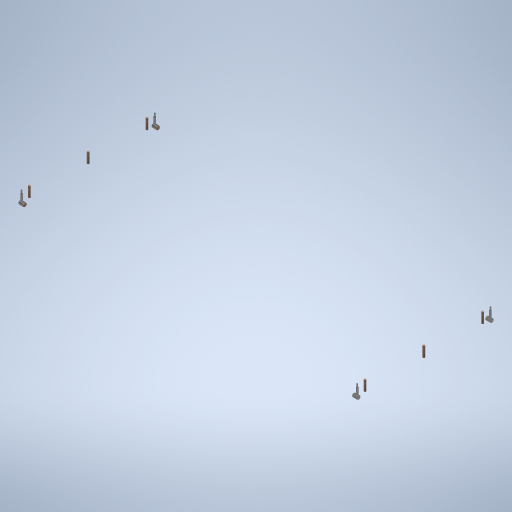
# Autodesk Inventor part: Minifixes pull Top Board-01
Saved by Autodesk Inventor 2024.3 (Build 283343000, 343)
## iProperties
RuleStatus: InUse
Created: 2014-05-13
Part Number: Minifixes pull Top Board-01
Material: Generic
Document SubType Name: Modeling
Designer: SauliusD
Density: 1 g/cm^3
Appearance: Default
Description: Minifixes pull Top Board
AfterDocNew0: Fire Form
Author: SauliusD
Autodesk Inventor part; units mm, degrees
ref_plane "XY Plane" through (0, 0, 0) normal (0, 0, 1) x (1, 0, 0)
sketch "Sketch1" plane through (0, 0, 0) normal (0, 0, 1) x (1, 0, 0)
  line L0 (-198.9585, 723.2553) -> (1147.0415, 723.2553)
  line L1 (1147.0415, 723.2553) -> (1147.0415, 177.2553)
  line L2 (1147.0415, 177.2553) -> (-198.9585, 177.2553)
  line L3 (-198.9585, 177.2553) -> (-198.9585, 723.2553)
  point P0 (0, 0)
  point P1 (474.0415, 177.2553)
  point P2 (-198.9585, 450.2553)
  constraints: 8 end point, 2 midpoint, 2 parallel, 1 horizontal, 1 perpendicular
ref_plane "Work Plane2" through (474.0415, 177.2553, 0) normal (1, 0, 0) x (0, 1, 0)
ref_plane "Work Plane3" through (-198.9585, 450.2553, 0) normal (0, 1, 0) x (-1, 0, 0)
sketch "Sketch3" plane through (0, 0, 0) normal (0, 0, 1) x (1, 0, 0)
  line L0 (-198.9585, 177.2553) -> (-198.9585, 723.2553) construction
  line L1 (-491.2585, 450.2553) -> (1439.3415, 450.2553) construction
  line L2 (474.0415, 897.0092) -> (474.0415, -298.2679) construction
  circle A0 centre (-211.4585, 178.2553) radius 4
  circle A1 centre (-211.4585, 210.2553) radius 4
  circle A2 centre (-211.4585, 722.2553) radius 4
  circle A3 centre (-211.4585, 690.2553) radius 4
  circle A4 centre (1159.5415, 178.2553) radius 4
  circle A5 centre (1159.5415, 210.2553) radius 4
  circle A6 centre (1159.5415, 722.2553) radius 4
  circle A7 centre (1159.5415, 690.2553) radius 4
  line L3 (-211.4585, -51.418) -> (-211.4585, -127.514) construction
  point P0 (0, 0)
  dimension "Between_Axis" = 546
  dimension "Dowel_D" = 8
  dimension "d9" = 32
  dimension "d10" = 544
  dimension "d29" = 12.5
  constraints: 8 centre point, 6 symmetric about line, 2 end point, 2 point on line, 1 equal radius, 1 parallel, 6 other
  measures "Between_Axis" distance of L0.start L0.end
  measures "Dowel_D" diameter of A0
  measures "d9" distance of A1.centre A0.centre
  measures "d10" distance of A2.centre A0.centre
  measures "d29" distance between parallel lines of L0 L3
extrude "Extrusion1" add sketch "Sketch3" against normal blind 34 contours A0 | A2 | A4 | A6
extrude "Extrusion2" add sketch "Sketch3" against normal blind 30 contours A1 | A3 | A5 | A7
extrude "Extrusion3" add sketch "Sketch3" along normal blind 12 contours A1 | A3 | A5 | A7
ref_plane "Work Plane4" through (-211.4585, -51.418, 0) normal (1, 0, 0) x (0, -1, 0)
sketch "Sketch4" plane through (-211.4585, -51.418, 0) normal (1, 0, 0) x (0, -1, 0)
  line L0 (-225.6733, 34) -> (-233.6733, 34) construction
  circle A0 centre (-229.6733, 34) radius 7.5
  point P0 (-51.418, 0)
  dimension "d18" = 15
  constraints: 1 centre point, 1 midpoint
  measures "d18" diameter of A0
extrude "Extrusion4" add sketch "Sketch4" along normal blind 12.5
extrude "Extrusion5" add sketch "Sketch4" against normal blind 6
mirror "Mirror1" about plane through (-198.9585, 450.2553, 0) normal (0, 1, 0) of "Extrusion4", "Extrusion5"
mirror "Mirror2" about plane through (474.0415, 177.2553, 0) normal (1, 0, 0) of "Extrusion4", "Extrusion5", "Mirror1"
sketch "Sketch5" plane through (0, 0, 0) normal (0, 0, 1) x (1, 0, 0)
  circle A0 centre (-211.4585, 178.2553) radius 4 projected
  circle A1 centre (-211.4585, 178.2553) radius 2.5
  point P0 (0, 0)
  dimension "d23" = 5
  constraints: 1 centre point
  measures "d23" diameter of A1
extrude "Extrusion6" add sketch "Sketch5" along normal up to surface (12 mm away) contours A1
mirror "Mirror3" about plane through (-198.9585, 450.2553, 0) normal (0, 1, 0) of "Extrusion6"
mirror "Mirror4" about plane through (474.0415, 177.2553, 0) normal (1, 0, 0) of "Extrusion6", "Mirror3"
sketch "Sketch6" plane through (0, 0, 0) normal (0, 0, 1) x (1, 0, 0)
  line L0 (-491.2585, 450.2553) -> (1439.3415, 450.2553) construction
  line L1 (474.0415, 867.9064) -> (474.0415, -144.6511) construction
  circle A0 centre (-211.4585, 450.2553) radius 4
  line L2 (-211.4585, 867.9064) -> (-211.4585, -144.6511) construction
  circle A1 centre (1159.5415, 450.2553) radius 4
  point P0 (0, 0)
  dimension "d26" = 8
  constraints: 2 centre point, 2 point on line, 1 symmetric about line, 1 other
  measures "d26" diameter of A0
extrude "Center Dowel Extrude" add sketch "Sketch6" against normal up to surface (42 mm away) from surface at 12
sketch "Sketch7" plane through (-198.9585, 178.2553, -34) normal (1, 0, 0) x (0, 0, -1)
  circle A0 centre (0, 0) radius 7.5 projected
  point P0 (-34, -178.2553)
extrude "Cap Extrude" add sketch "Sketch7" along normal blind 2 separate body
fillet "Cap Fillet" radius 1.6 1 edges at (-196.9585, 178.2553, -26.5)
mirror "Cap Mirror" about plane through (-198.9585, 450.2553, 0) normal (0, 1, 0) of "Cap Extrude", "Cap Fillet" bodies 2
mirror "Cap Mirror2" about plane through (474.0415, 177.2553, 0) normal (1, 0, 0) of "Cap Extrude", "Cap Fillet", "Cap Mirror" bodies 2
equation "\"d9\" = Step"
equation "\"d10\" = Between_Minifixes"
equation "\"d29\" = Board_Half_T"
equation "\"d26\" = Dowel_D"
equation "\"Step\" = 32"
equation "\"Between_Minifixes\" = 544"
equation "\"Board_Half_T\" = 12.5"
